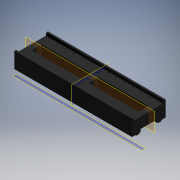
# Autodesk Inventor part: socket
Saved by Autodesk Inventor 2018 (Build 220112000, 112)
## iProperties
Created: 2017-04-13
Part Number: socket
Material: Acetal Resin, Black
Document SubType Name: Modeling
Designer: kampe_000
Density: 1.425 g/cm^3
Appearance: Smooth - Black
Author: kampe_000
Autodesk Inventor part; units mm, degrees
ref_plane "YZ Plane" through (0, 0, 0) normal (1, 0, 0) x (0, 1, 0)
ref_plane "XZ Plane" through (0, 0, 0) normal (0, 1, 0) x (-1, 0, 0)
sketch "Sketch1" plane through (0, 0, 0) normal (0, 1, 0) x (-1, 0, 0)
  line L0 (0, 0) -> (-35.56, 0)
  line L1 (-35.56, 0) -> (-35.56, -10.16)
  line L2 (-35.56, -10.16) -> (0, -10.16)
  line L3 (0, -10.16) -> (0, 0)
  dimension "d0" = 35.56
  dimension "d1" = 10.16
  constraints: 8 end point, 2 parallel, 1 horizontal, 1 perpendicular
  measures "d0" distance of L2.end L1.end
  measures "d1" distance of L1.end L0.end
extrude "Extrusion1" add sketch "Sketch1" along normal blind 5.1
sketch "Sketch2" plane through (35.56, 0, 0) normal (1, 0, 0) x (0, 0, -1)
  line L0 (0, 0) -> (0, 5.1) projected
  line L1 (0, 0.3) -> (10.16, 0.3) construction
  line L2 (10.16, 0) -> (10.16, 5.1) projected
  line L3 (0, 0) -> (10.16, 0) projected
  line L4 (0, 5.1) -> (10.16, 5.1) projected
  line L5 (5.08, 5.1) -> (5.08, 0) construction
  line L6 (5.08, 0.3) -> (1.27, 0.3) construction
  line L7 (1.27, 0.3) -> (0, 0.3)
  line L8 (0, 0.3) -> (0, 0)
  line L9 (0, 0) -> (1.27, 0)
  line L10 (1.27, 0) -> (1.27, 0.3)
  line L11 (8.89, 0.3) -> (10.16, 0.3)
  line L12 (10.16, 0.3) -> (10.16, 0)
  line L13 (10.16, 0) -> (8.89, 0)
  line L14 (8.89, 0) -> (8.89, 0.3)
  line L15 (2.27, 0.3) -> (7.89, 0.3)
  line L16 (7.89, 0.3) -> (7.89, 0)
  line L17 (7.89, 0) -> (2.27, 0)
  line L18 (2.27, 0) -> (2.27, 0.3)
  dimension "d4" = 0.3
  dimension "d5" = 3.81
  dimension "d6" = 1
  dimension "d7" = 1
  constraints: 30 end point, 6 point on line, 4 parallel, 4 symmetric about line, 3 horizontal, 3 midpoint, 2 perpendicular
  measures "d4" distance between parallel lines of L1 L3
  measures "d5" distance of L6.start L6.end
  measures "d6" distance between parallel lines of L18 L10
  measures "d7" distance between parallel lines of L14 L16
extrude "Extrusion2" cut sketch "Sketch2" against normal through all contours L0 L7 L10 L3 | L18 L15 L16 L3 | L2 L3 L14 L11
sketch "Sketch3" plane through (35.56, 5.1, 0) normal (1, 0, 0) x (0, 0, -1)
  line L0 (2.67, -4.8) -> (7.49, -4.8)
  line L1 (7.49, -4.8) -> (7.49, -4)
  line L2 (7.49, -4) -> (2.67, -4)
  line L3 (2.67, -4) -> (2.67, -4.8)
  line L4 (2.27, -5.1) -> (2.27, -4.8) projected
  line L5 (7.89, -4.8) -> (7.89, -5.1) projected
  point P0 (0, -5.1)
  dimension "d12" = 0.4
  dimension "d13" = 0.4
  dimension "d14" = 0.8
  constraints: 8 end point, 2 parallel, 1 horizontal, 1 perpendicular
  measures "d12" distance between parallel lines of L3 L4
  measures "d13" distance between parallel lines of L5 L1
  measures "d14" distance between parallel lines of L0 L2
extrude "Extrusion3" cut sketch "Sketch3" against normal through all
sketch "Sketch4" plane through (35.56, 5.1, 0) normal (1, 0, 0) x (0, 0, -1)
  line L0 (0, 0) -> (10.16, 0) projected
  line L1 (0.5, 0) -> (0.6411, -0.8)
  line L2 (0.6411, -0.8) -> (9.5189, -0.8)
  line L3 (9.5189, -0.8) -> (9.66, 0)
  line L4 (0.5, 0) -> (9.66, 0)
  point P0 (0, -5.1)
  dimension "d15" = 0.5
  dimension "d16" = 0.5
  dimension "d17" = 0.8
  dimension "d18" = 100
  dimension "d19" = 100
  constraints: 8 end point, 4 point on line, 1 parallel
  measures "d15" distance of L1.start L0.start
  measures "d16" distance of L0.end L3.end
  measures "d17" distance between parallel lines of L0 L2
  measures "d18" angle of L2 L1
  measures "d19" angle of L2 L3
extrude "Extrusion4" cut sketch "Sketch4" against normal through all
sketch "Sketch5" plane through (35.56, 4.3, -0.6411) normal (0, 1, 0) x (1, 0, 0)
  line L0 (0, 9.5189) -> (-35.56, 9.5189) projected
  line L1 (-17.78, 9.5189) -> (-17.78, -0.6411) construction
  line L2 (-35.56, -0.6411) -> (0, -0.6411) projected
  line L3 (-35.56, 0) -> (-35.56, 8.8779) projected
  line L4 (-35.56, 4.4389) -> (0, 4.4389) construction
  line L5 (0, 2.0289) -> (0, 6.8489) projected
  line L6 (-33.88, 2.9389) -> (-18.88, 2.9389)
  line L7 (-18.88, 2.9389) -> (-18.88, 5.9389)
  line L8 (-18.88, 5.9389) -> (-33.88, 5.9389)
  line L9 (-33.88, 5.9389) -> (-33.88, 2.9389)
  line L10 (-33.88, 2.9389) -> (-18.88, 5.9389) construction
  line L11 (-18.88, 2.9389) -> (-33.88, 5.9389) construction
  line L12 (-1.68, 2.9389) -> (-16.68, 2.9389)
  line L13 (-16.68, 2.9389) -> (-16.68, 5.9389)
  line L14 (-16.68, 5.9389) -> (-1.68, 5.9389)
  line L15 (-1.68, 5.9389) -> (-1.68, 2.9389)
  line L16 (-1.68, 2.9389) -> (-16.68, 5.9389) construction
  line L17 (-16.68, 2.9389) -> (-1.68, 5.9389) construction
  point P0 (-26.38, 4.4389)
  point P1 (-9.18, 4.4389)
  dimension "d22" = 15
  dimension "d23" = 3
  dimension "d24" = 8.6
  constraints: 28 end point, 8 midpoint, 5 symmetric about line, 2 parallel, 1 horizontal, 1 perpendicular, 1 point on line
  measures "d22" distance of L8.end L7.end
  measures "d23" distance of L7.end L6.end
  measures "d24" distance from line of L1 point (-26.38, 4.439)
extrude "Extrusion5" cut sketch "Sketch5" against normal through all
ref_plane "Work Plane2" through (0, 5.1, -1.27) normal (0, 0, 1) x (1, 0, 0)
ref_plane "Work Plane1" through (0, 5.1, -5.08) normal (0, 0, 1) x (1, 0, 0)
ref_plane "Work Plane3" through (0, -3, 0) normal (0, -1, 0) x (1, 0, 0)
ref_plane "Work Plane4" through (17.78, 0, -8.89) normal (-1, 0, 0) x (0, 0, 1)
sketch "Sketch7" plane through (35.56, 0.3, -1.27) normal (0, -1, 0) x (1, 0, 0)
  line L0 (-34.29, 0) -> (-1.27, 0)
  line L1 (-17.78, -10.922) -> (-17.78, 3.302) projected
  line L2 (-42.672, -3.81) -> (7.112, -3.81) projected
  line L3 (-0.97, 0) -> (-1.57, 0)
  line L4 (-1.57, 0) -> (-1.57, 0.15)
  line L5 (-1.57, 0.15) -> (-0.97, 0.15)
  line L6 (-0.97, 0.15) -> (-0.97, 0)
  line L7 (-0.97, 0) -> (-1.57, 0.15) construction
  line L8 (-1.57, 0) -> (-0.97, 0.15) construction
  point P0 (-35.56, 1.27)
  point P1 (-1.27, 0)
  point P2 (-1.27, 0.075)
  dimension "d29" = 33.02
  dimension "d30" = 3.81
  dimension "d31" = 0.6
  dimension "d32" = 0.15
  constraints: 14 end point, 3 midpoint, 2 horizontal, 2 parallel, 1 coincident, 1 perpendicular, 1 symmetric about line
  measures "d29" distance of L0.end L0.start
  measures "d30" distance between parallel lines of L2 L0
  measures "d31" distance of L4.end L5.end
  measures "d32" distance of L3.end L4.end
extrude "Extrusion6" cut sketch "Sketch7" against normal through all
pattern_linear "Rectangular Pattern1" count 14 spacing 2.54 along (-1, 0, 0) count 2 spacing 7.92 along (0, 0, -1) of "Extrusion6"
equation "\"d7\" = d6"
equation "\"d13\" = d12"
equation "\"d16\" = d15"
body "Solid1"
